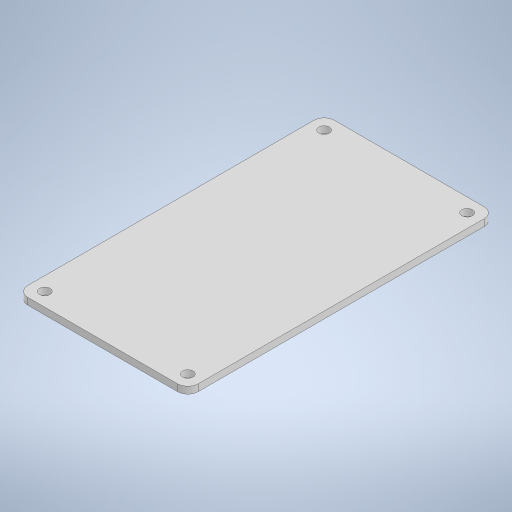
# Autodesk Inventor part: контур
Saved by Autodesk Inventor 2023.1 (Build 271208000, 208)
## iProperties
Created: 2025-01-21
Part Number: контур
Material: Типовые
Document SubType Name: Modeling
Designer: DELL
Density: 1 g/cm^3
Appearance: По умолчанию
Author: DELL
Autodesk Inventor part; units mm, degrees
ref_plane "YZ Plane" through (0, 0, 0) normal (1, 0, 0) x (0, 1, 0)
ref_plane "XZ Plane" through (0, 0, 0) normal (0, 1, 0) x (-1, 0, 0)
ref_plane "XY Plane" through (0, 0, 0) normal (0, 0, 1) x (1, 0, 0)
sketch "Эскиз8" plane through (0, 0, 0) normal (0, 1, 0) x (-1, 0, 0)
  line L0 (11.8002, -55.25) -> (55.8002, -55.25)
  line L1 (58.8002, -52.25) -> (58.8002, 31.75)
  line L2 (55.8002, 34.75) -> (11.8002, 34.75)
  line L3 (8.8002, 31.75) -> (8.8002, -52.25)
  arc A0 (11.8002, 34.75) -> (8.8002, 31.75) centre (11.8002, 31.75) ccw
  arc A1 (8.8002, -52.25) -> (11.8002, -55.25) centre (11.8002, -52.25) ccw
  arc A2 (55.8002, -55.25) -> (58.8002, -52.25) centre (55.8002, -52.25) ccw
  arc A3 (58.8002, 31.75) -> (55.8002, 34.75) centre (55.8002, 31.75) ccw
  line L4 (12.8002, 30.75) -> (54.8002, 30.75) construction
  line L5 (54.8002, 30.75) -> (54.8002, -51.25) construction
  line L6 (54.8002, -51.25) -> (12.8002, -51.25) construction
  line L7 (12.8002, -51.25) -> (12.8002, 30.75) construction
  circle A4 centre (54.8002, 30.75) radius 1.575
  circle A5 centre (12.8002, 30.75) radius 1.575
  circle A6 centre (54.8002, -51.25) radius 1.575
  circle A7 centre (12.8002, -51.25) radius 1.575
  point P0 (0, 0)
  point P1 (8.8002, -55.25)
  point P2 (58.8002, 34.75)
  point P3 (58.8002, -55.25)
  point P4 (8.8002, 34.75)
  dimension "d54" = 50
  dimension "d55" = 90
  dimension "d56" = 3
  dimension "d57" = 4
  dimension "d58" = 3.15
  dimension "d59" = 3.15
  dimension "d60" = 3.15
  dimension "d61" = 3.15
  constraints: 16 end point, 8 centre point, 8 point on circle, 8 point on line, 8 tangent, 4 coincident, 4 parallel, 3 equal radius, 2 perpendicular, 1 horizontal, 3 other
  measures "d54" distance of point (8.8, 34.75) point (58.8, 34.75)
  measures "d55" distance of point (58.8, 34.75) point (58.8, -55.25)
  measures "d56" radius of A0
  measures "d57" distance between parallel lines of L2 L4
  measures "d58" diameter of A4
  measures "d59" diameter of A5
  measures "d60" diameter of A6
  measures "d61" diameter of A7
extrude "Выдавливание6" add sketch "Эскиз8" along normal blind 2
